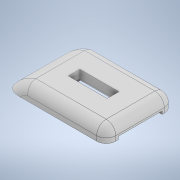
# Autodesk Inventor part: Case - Top
Saved by Autodesk Inventor 2020 (Build 240168000, 168)
## iProperties
Created: 2019-07-11
Part Number: Case - Top
Material: Generic
Document SubType Name: Modeling
Designer: tyrre
Density: 1 g/cm^3
Appearance: Default
Author: tyrre
Autodesk Inventor part; units mm, degrees
ref_plane "YZ Plane" through (0, 0, 0) normal (1, 0, 0) x (0, 1, 0)
ref_plane "XZ Plane" through (0, 0, 0) normal (0, 1, 0) x (-1, 0, 0)
ref_plane "XY Plane" through (0, 0, 0) normal (0, 0, 1) x (1, 0, 0)
sketch "Sketch1" plane through (0, 0, 0) normal (0, 0, 1) x (1, 0, 0)
  line L0 (-20.935, 3.75) -> (20.935, 3.75)
  line L1 (20.935, 3.75) -> (20.935, -3.75)
  line L2 (20.935, -3.75) -> (-20.935, -3.75)
  line L3 (-20.935, -3.75) -> (-20.935, 3.75)
  line L4 (-20.935, 3.75) -> (20.935, -3.75) construction
  line L5 (20.935, 3.75) -> (-20.935, -3.75) construction
  point P0 (0, 0)
  dimension "d0" = 41.87
  dimension "d1" = 7.5
  constraints: 12 end point, 2 midpoint, 2 parallel, 1 horizontal, 1 perpendicular
  measures "d0" distance of L1.end L2.end
  measures "d1" distance of L0.end L1.end
extrude "Extrusion1" add sketch "Sketch1" along normal mid plane 35.5
sketch "Sketch2" plane through (-20.935, -3.75, 17.75) normal (0, -1, 0) x (1, 0, 0)
  line L0 (0, -35.5) -> (0, 0) projected
  line L1 (0, -35.5) -> (0, -29.307)
  line L2 (0, -29.307) -> (5, -29.307)
  line L3 (5, -29.307) -> (5, -6.193)
  line L4 (5, -6.193) -> (41.87, -6.193)
  line L5 (41.87, -6.193) -> (41.87, -29.307)
  line L6 (41.87, -29.307) -> (5, -29.307)
  point P0 (20.935, -17.75)
  dimension "d4" = 6.193
  dimension "d5" = 5
  dimension "d6" = 23.114
  dimension "d7" = 36.87
  constraints: 12 end point, 3 perpendicular, 2 parallel, 1 point on line
  measures "d4" distance of L0.start L1.end
  measures "d5" distance of L1.end L2.end
  measures "d6" distance of L2.end L3.end
  measures "d7" distance of L3.end L4.end
extrude "Extrusion2" cut sketch "Sketch2" against normal blind 1.6
sketch "Sketch3" plane through (-20.935, -2.15, 17.75) normal (0, -1, 0) x (1, 0, 0)
  line L0 (5, -29.307) -> (5, -6.193) projected
  line L1 (5, -29.307) -> (5, -21.75)
  line L2 (5, -21.75) -> (5, -13.75)
  line L3 (5, -13.75) -> (40, -13.75)
  line L4 (40, -13.75) -> (40, -21.75)
  line L5 (40, -21.75) -> (5, -21.75)
  point P0 (20.935, -17.75)
  dimension "d10" = 7.557
  dimension "d11" = 8
  dimension "d12" = 35
  constraints: 10 end point, 2 parallel, 2 point on line, 1 perpendicular
  measures "d10" distance of L0.start L1.end
  measures "d11" distance of L1.end L2.end
  measures "d12" distance of L2.end L3.end
extrude "Extrusion3" cut sketch "Sketch3" against normal blind 1.6
fillet "Fillet1" radius 5 2 edges at (0, 3.75, 17.75) (0, 3.75, -17.75)
fillet "Fillet2" radius 5 5 edges at (20.935, 2.2855, -16.2855) (20.935, -2.5, -17.75) (20.935, 2.2855, 16.2855) (20.935, -2.5, 17.75) (20.935, 3.75, 0)
sketch "Sketch5" plane through (-20.935, -0.55, 17.75) normal (0, -1, 0) x (1, 0, 0)
  line L0 (5, -29.307) -> (5, -21.75) projected
  line L1 (5, -21.75) -> (5, -20.85)
  line L2 (5, -29.307) -> (5, -6.193) projected
  line L3 (5, -20.85) -> (7.25, -20.85)
  line L4 (7.25, -20.85) -> (7.25, -14.65)
  line L5 (7.25, -14.65) -> (27.75, -14.65)
  line L6 (27.75, -14.65) -> (27.75, -20.85)
  line L7 (27.75, -20.85) -> (7.25, -20.85)
  point P0 (20.935, -17.75)
  dimension "d22" = 0.9
  dimension "d23" = 2.25
  dimension "d24" = 6.2
  dimension "d25" = 20.5
  constraints: 12 end point, 2 parallel, 1 horizontal, 1 perpendicular, 1 point on line, 1 vertical
  measures "d22" distance of L0.end L1.end
  measures "d23" distance of L1.end L3.end
  measures "d24" distance of L3.end L4.end
  measures "d25" distance of L4.end L5.end
extrude "Extrusion5" cut sketch "Sketch5" against normal through all
sketch "Sketch6" plane through (-20.935, -3.75, -17.75) normal (0, -1, 0) x (1, 0, 0)
  line L0 (0, 0) -> (0, 35.5) projected
  line L1 (0, 35.5) -> (-15, 35.5)
  line L2 (-15, 35.5) -> (-15, 0)
  line L3 (-15, 0) -> (0, 0)
  line L4 (0, 0) -> (0, 35.5)
  point P0 (20.935, 17.75)
  dimension "d28" = 15
  dimension "d29" = 35.5
  constraints: 8 end point, 2 parallel, 1 horizontal, 1 perpendicular
  measures "d28" distance of L3.end L2.end
  measures "d29" distance of L2.end L1.end
extrude "Extrusion6" add sketch "Sketch6" against normal blind 7.5
fillet "Fillet3" [suppressed]
sketch "Sketch7" plane through (0, 0, 17.75) normal (0, 0, 1) x (1, 0, 0)
  line L0 (-20.9589, -1.4001) -> (-20.9589, -3.75)
  line L1 (15.935, -3.75) -> (-35.935, -3.75) projected
  line L2 (-35.935, -3.75) -> (-20.9589, -3.75)
  line L3 (-20.9589, -3.75) -> (-20.9589, -14.15)
  line L4 (-20.9589, -14.15) -> (-35.935, -14.15)
  line L5 (-35.935, -14.15) -> (-35.935, -3.75)
  point P0 (0, 0)
  dimension "d33" = 10.4
  constraints: 10 end point, 2 parallel, 1 horizontal, 1 perpendicular, 1 point on line, 1 vertical
  measures "d33" distance of L0.end L3.end
extrude "Extrusion7" add sketch "Sketch7" against normal blind 35.5
sketch "Sketch8" plane through (0, 0, 17.75) normal (0, 0, 1) x (1, 0, 0)
  line L0 (-35.935, 3.75) -> (-35.935, -14.15) projected
  line L1 (-35.935, 3.75) -> (-20.935, 3.75) projected
  arc A0 (-20.935, 3.75) -> (-35.935, -14.15) centre (-14.1441, -17.1757) ccw
  line L2 (-35.935, -14.15) -> (-35.935, 3.75)
  point P0 (0, 0)
  dimension "d36" = 22
  constraints: 2 end point, 2 point on circle, 1 centre point, 1 collinear
  measures "d36" radius of A0
extrude "Extrusion8" cut sketch "Sketch8" against normal through all
sketch "Sketch9" plane through (0, 0, 17.75) normal (0, 0, 1) x (1, 0, 0)
  line L0 (-20.9589, -3.75) -> (-20.9589, -14.15) projected
  line L1 (-20.9589, -3.75) -> (-37.0076, -3.75)
  line L2 (-37.0076, -3.75) -> (-37.0076, -16.8891)
  line L3 (-37.0076, -16.8891) -> (-20.9589, -16.8891)
  line L4 (-20.9589, -16.8891) -> (-20.9589, -3.75)
  point P0 (0, 0)
  constraints: 8 end point, 2 parallel, 2 perpendicular
extrude "Extrusion9" cut sketch "Sketch9" against normal through all
fillet "Fillet4" radius 5 2 edges at (-26.8211, 0.8047, 17.75) (-26.8211, 0.8047, -17.75)
body "Solid1"
